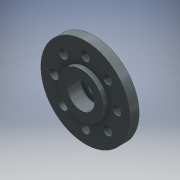
# Autodesk Inventor part: ServoHorn
Saved by Autodesk Inventor 2016 (Build 200138000, 138)
## iProperties
Created: 2015-09-12
Part Number: ServoHorn
Material: 一般
Document SubType Name: Modeling
Designer: daisuke
Density: 1 g/cm^3
Appearance: 鉄 灰色
Author: daisuke
Autodesk Inventor part; units mm, degrees
ref_plane "YZ Plane" through (0, 0, 0) normal (1, 0, 0) x (0, 1, 0)
ref_plane "XZ Plane" through (0, 0, 0) normal (0, 1, 0) x (-1, 0, 0)
ref_plane "XY Plane" through (0, 0, 0) normal (0, 0, 1) x (1, 0, 0)
sketch "スケッチ1" plane through (0, 0, 0) normal (0, 1, 0) x (-1, 0, 0)
  circle A0 centre (0, 0) radius 10
  circle A1 centre (0, 0) radius 7 construction
  circle A2 centre (-7, 0) radius 1
  circle A3 centre (-4.9497, -4.9497) radius 1
  circle A4 centre (4.9497, -4.9497) radius 1
  circle A5 centre (0, -7) radius 1
  circle A6 centre (7, 0) radius 1
  circle A7 centre (4.9497, 4.9497) radius 1
  circle A8 centre (0, 7) radius 1
  circle A9 centre (-4.9497, 4.9497) radius 1
  circle A10 centre (0, 0) radius 5
  dimension "d26" = 14
  dimension "d0" = 20
  dimension "d27" = 2
  dimension "d28" = 2
  dimension "d29" = 2
  dimension "d30" = 2
  dimension "d31" = 2
  dimension "d32" = 2
  dimension "d33" = 2
  dimension "d34" = 2
  dimension "d35" = 10
  constraints: 10 centre point, 3 coincident, 1 horizontal alignment, 2 other
  measures "d0" diameter of A0
  measures "d27" diameter of A2
  measures "d28" diameter of A3
  measures "d29" diameter of A5
  measures "d30" diameter of A4
  measures "d31" diameter of A6
  measures "d32" diameter of A7
  measures "d33" diameter of A8
  measures "d34" diameter of A9
  measures "d35" diameter of A10
extrude "押し出し1" add sketch "スケッチ1" along normal blind 2 contours A0 | A2 | A3 | A4 | A5 | A6 | A7 | A8 | A9 | A10
sketch "スケッチ2" plane through (0, 2, 0) normal (0, 1, 0) x (1, 0, 0)
  circle A0 centre (0, 0) radius 7 construction
  circle A1 centre (-7, 0) radius 1
  circle A2 centre (-4.9497, -4.9497) radius 1
  circle A3 centre (0, -7) radius 1
  circle A4 centre (4.9497, -4.9497) radius 1
  circle A5 centre (7, 0) radius 1
  circle A6 centre (4.9497, 4.9497) radius 1
  circle A7 centre (-4.9497, 4.9497) radius 1
  circle A8 centre (0, 7) radius 1
  dimension "d3" = 14
  dimension "d4" = 2
  dimension "d5" = 2
  dimension "d6" = 2
  dimension "d7" = 2
  dimension "d8" = 2
  dimension "d9" = 2
  dimension "d10" = 2
  dimension "d11" = 2
  constraints: 8 centre point, 1 coincident, 1 horizontal alignment, 2 other
  measures "d4" diameter of A1
  measures "d5" diameter of A2
  measures "d6" diameter of A3
  measures "d7" diameter of A4
  measures "d8" diameter of A5
  measures "d9" diameter of A6
  measures "d10" diameter of A8
  measures "d11" diameter of A7
extrude "押し出し2" cut sketch "スケッチ2" against normal blind 2
sketch "スケッチ3" plane through (0, 2, 0) normal (0, 1, 0) x (1, 0, 0)
  circle A0 centre (0, 0) radius 5
  dimension "d14" = 10
  constraints: 1 centre point, 1 coincident
  measures "d14" diameter of A0
extrude "押し出し3" add sketch "スケッチ3" along normal blind 1
sketch "スケッチ4" plane through (0, 3, 0) normal (0, 1, 0) x (1, 0, 0)
  circle A0 centre (0, 0) radius 1.6
  dimension "d17" = 3.2
  constraints: 1 centre point, 1 coincident
  measures "d17" diameter of A0
extrude "押し出し4" cut sketch "スケッチ4" against normal blind 1
sketch "スケッチ5" plane through (0, 0, 0) normal (0, -1, 0) x (1, 0, 0)
  circle A0 centre (0, 0) radius 5
  dimension "d20" = 10
  constraints: 1 centre point, 1 coincident
  measures "d20" diameter of A0
extrude "押し出し5" add sketch "スケッチ5" along normal blind 1
sketch "スケッチ6" plane through (0, -1, 0) normal (0, -1, 0) x (1, 0, 0)
  circle A0 centre (0, 0) radius 3
  dimension "d23" = 6
  constraints: 1 centre point, 1 coincident
  measures "d23" diameter of A0
extrude "押し出し6" cut sketch "スケッチ6" against normal blind 3
